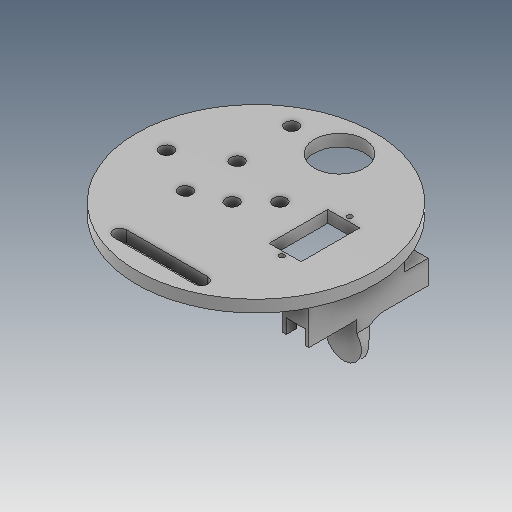
# Autodesk Inventor part: EndEffectorPlate
Saved by Autodesk Inventor 2020.3 (Build 243373000, 373)
## iProperties
Created: 2021-08-11
Part Number: EndEffectorPlate
Material: ABS Plastic
Document SubType Name: Modeling
Designer: justi
Density: 1.06 g/cm^3
Appearance: Smooth - Medium Gray
Mass: 42.5954 g
Surface Area: 204.332 cm^2
Volume: 40.1844 cm^3
Author: justi
Autodesk Inventor part; units mm, degrees
ref_plane "YZ Plane" through (0, 0, 0) normal (1, 0, 0) x (0, 1, 0)
ref_plane "XZ Plane" through (0, 0, 0) normal (0, 1, 0) x (-1, 0, 0)
ref_plane "XY Plane" through (0, 0, 0) normal (0, 0, 1) x (1, 0, 0)
sketch "Sketch1" plane through (0, 0, 0) normal (0, 1, 0) x (-1, 0, 0)
  circle A0 centre (0, 0) radius 50
  dimension "d0" = 100
  constraints: 1 centre point, 1 coincident
  measures "d0" diameter of A0
extrude "Extrusion1" add sketch "Sketch1" along normal mid plane 5
sketch "Sketch2" plane through (0, 2.5, 0) normal (0, 1, 0) x (1, 0, 0)
  line L0 (-5, 5) -> (5, 5) construction
  line L1 (5, 5) -> (5, -5) construction
  line L2 (5, -5) -> (-5, -5) construction
  line L3 (-5, -5) -> (-5, 5) construction
  line L4 (-5, 5) -> (5, -5) construction
  line L5 (5, 5) -> (-5, -5) construction
  circle A0 centre (5, 5) radius 2.75
  circle A1 centre (-5, -5) radius 2.75
  point P0 (0, 0)
  dimension "d77" = 10
  dimension "d78" = 10
  dimension "d80" = 5.5
  dimension "d81" = 5.5
  constraints: 12 end point, 2 centre point, 2 coincident, 2 midpoint, 2 parallel, 1 horizontal, 1 perpendicular
  measures "d77" distance of L1.end L2.end
  measures "d78" distance of L0.end L1.end
  measures "d80" diameter of A0
  measures "d81" diameter of A1
extrude "Extrusion2" cut sketch "Sketch2" against normal blind 10
sketch "Sketch3" plane through (0, 2.5, 0) normal (0, 1, 0) x (1, 0, 0)
  line L0 (0, 0) -> (25, 0) construction
  line L1 (18.8, -11.3) -> (31.2, -11.3)
  line L2 (31.2, -11.3) -> (31.2, 11.3)
  line L3 (31.2, 11.3) -> (18.8, 11.3)
  line L4 (18.8, 11.3) -> (18.8, -11.3)
  line L5 (18.8, -11.3) -> (31.2, 11.3) construction
  line L6 (31.2, -11.3) -> (18.8, 11.3) construction
  line L7 (25, 0) -> (25, 14.25) construction
  line L8 (25, 0) -> (25, -14.25) construction
  circle A0 centre (25, 14.25) radius 1.1
  circle A1 centre (25, -14.25) radius 1.1
  dimension "d9" = 25
  dimension "d10" = 12.4
  dimension "d11" = 22.6
  dimension "d21" = 14.25
  dimension "d22" = 14.25
  dimension "d23" = 2.2
  dimension "d24" = 2.2
  constraints: 18 end point, 2 centre point, 2 coincident, 2 horizontal, 2 midpoint, 2 parallel, 2 vertical, 1 perpendicular
  measures "d9" distance of L0.start L0.end
  measures "d10" distance of L3.end L2.end
  measures "d11" distance of L2.end L1.end
  measures "d21" distance of L0.end L7.end
  measures "d22" distance of L0.end L8.end
  measures "d23" diameter of A0
  measures "d24" diameter of A1
extrude "Extrusion3" cut sketch "Sketch3" against normal blind 10
sketch "Sketch5" plane through (0, -2.5, 0) normal (0, -1, 0) x (1, 0, 0)
  line L0 (31.2, -11.3) -> (33.7, -11.3)
  line L1 (33.7, -11.3) -> (33.7, 11.3)
  line L2 (33.7, 11.3) -> (31.2, 11.3)
  line L3 (31.2, 11.3) -> (31.2, -11.3)
  line L4 (31.2, -11.3) -> (31.2, 11.3) construction
  line L5 (31.2, 0) -> (39.7, 0) construction
  line L6 (39.7, 0) -> (39.7, -20) construction
  line L7 (39.7, -20) -> (31.2, -20)
  line L8 (31.2, -20) -> (31.2, 20)
  line L9 (31.2, 20) -> (39.7, 20)
  line L10 (39.7, 20) -> (39.7, -20)
  line L11 (33.7, -11.3) -> (33.7, -20)
  line L12 (33.7, 11.3) -> (33.7, 20)
  point P0 (0, 0)
  point P1 (31.2, 11.3)
  dimension "d34" = 2.5
  dimension "d35" = 8.5
  dimension "d36" = 20
  dimension "d37" = 40
  constraints: 24 end point, 4 parallel, 4 perpendicular, 3 horizontal, 2 point on line, 1 midpoint, 1 vertical
  measures "d34" distance of L2.end L1.end
  measures "d35" distance of L5.start L5.end
  measures "d36" distance of L5.end L6.end
  measures "d37" distance of L7.end L8.end
extrude "Extrusion5" add sketch "Sketch5" along normal blind 11.8 contours L1 L12 L9 L10 L7 L11
sketch "Sketch6" plane through (0, -2.5, 0) normal (0, -1, 0) x (1, 0, 0)
  line L0 (31.2, -11.3) -> (31.2, 11.3) projected
  line L1 (31.2, 0) -> (33.7, 0)
  line L2 (33.7, 0) -> (33.7, -20)
  line L3 (33.7, -20) -> (31.2, -20)
  line L4 (31.2, -20) -> (31.2, 0)
  line L5 (39.7, 20) -> (33.7, 20) projected
  line L6 (31.2, 0) -> (33.7, 0)
  line L7 (33.7, 0) -> (33.7, 20)
  line L8 (33.7, 20) -> (31.2, 20)
  line L9 (31.2, 20) -> (31.2, 0)
  line L10 (18.8, 11.3) -> (31.2, 11.3) projected
  line L11 (31.2, 11.3) -> (33.7, 11.3)
  line L12 (33.7, -20) -> (33.7, 20) projected
  line L13 (39.7, 20) -> (42.2, 20)
  line L14 (42.2, 20) -> (42.2, -20)
  line L15 (42.2, -20) -> (39.7, -20)
  line L16 (39.7, -20) -> (39.7, 20)
  line L17 (31.2, -15.9678) -> (33.7, -15.9678)
  point P0 (0, 0)
  point P1 (31.2, 11.3)
  dimension "d40" = 2.5
  constraints: 28 end point, 6 parallel, 5 perpendicular, 3 horizontal, 3 point on line, 1 midpoint
  measures "d40" distance of L14.end L15.end
extrude "Extrusion6" add sketch "Sketch6" along normal blind 16.8 contours L13 L14 L15 L16 | L17 L2 L3 L4 | L9 L8 L7 L11
sketch "Sketch7" plane through (0, -19.3, 0) normal (0, -1, 0) x (1, 0, 0)
  line L0 (42.2, -20) -> (31.2, -20) projected
  line L1 (31.2, -20) -> (42.2, -20)
  line L2 (42.2, -20) -> (42.2, 0)
  line L3 (42.2, 0) -> (31.2, 0)
  line L4 (31.2, 0) -> (31.2, -20)
  point P0 (0, 0)
  constraints: 8 end point, 2 parallel, 1 horizontal, 1 perpendicular
extrude "Extrusion7" add sketch "Sketch7" along normal blind 2.5
sketch "Sketch8" plane through (31.2, -19.3, 0) normal (0, 0, 1) x (1, 0, 0)
  line L0 (0, -2.5) -> (11, -2.5) construction
  line L1 (5.5, -2.5) -> (5.5, -10) construction
  circle A0 centre (5.5, -10) radius 7.5
  line L2 (0, 16.8) -> (0, -2.5) construction
  line L3 (11, 16.8) -> (11, -2.5) projected
  line L4 (11, -2.5) -> (11, -4.901)
  line L5 (0, -2.5) -> (0, -4.901)
  line L6 (11, -2.5) -> (0, -2.5)
  point P0 (-31.2, 19.3)
  dimension "d45" = 7.5
  constraints: 8 end point, 3 point on circle, 2 collinear, 1 centre point, 1 coincident, 1 midpoint, 1 parallel, 1 vertical
  measures "d45" distance of L1.start L1.end
extrude "Extrusion8" add sketch "Sketch8" against normal blind 3
fillet "Fillet1" radius 8.25 1 edges at (36.7, -21.8, -3)
sketch "Sketch9" plane through (42.2, -2.5, -20) normal (0, 0, -1) x (-1, 0, 0)
  line L0 (11, -16.8) -> (8.5, -16.8) projected
  line L1 (8.5, -16.8) -> (2.5, -16.8)
  line L2 (2.5, -16.8) -> (2.5, -11.8)
  line L3 (2.5, -11.8) -> (8.5, -11.8)
  line L4 (8.5, -11.8) -> (8.5, -16.8)
  line L5 (11, 0) -> (11, -19.3) projected
  line L6 (0, 0) -> (0, -19.3) projected
  line L7 (11, -19.3) -> (0, -19.3)
  line L8 (0, -19.3) -> (0, -9.35)
  line L9 (0, -9.35) -> (11, -9.35)
  line L10 (11, -9.35) -> (11, -19.3)
  point P0 (42.2, 2.5)
  dimension "d49" = 9.95
  constraints: 16 end point, 4 parallel, 2 horizontal, 2 perpendicular, 1 point on line
  measures "d49" distance of L7.end L8.end
extrude "Extrusion9" add sketch "Sketch9" along normal blind 10
sketch "Sketch12" plane through (0, 2.5, 0) normal (0, 1, 0) x (1, 0, 0)
  circle A0 centre (-25, 0) radius 12.5 construction
  line L0 (-25, 0) -> (-18.75, -10.8253) construction
  line L1 (-25, 0) -> (-37.5, 0) construction
  line L2 (-25, 0) -> (-18.75, 10.8253) construction
  circle A1 centre (-37.5, 0) radius 2.75
  circle A2 centre (-18.75, 10.8253) radius 2.75
  circle A3 centre (-18.75, -10.8253) radius 2.75
  point P0 (0, 0)
  dimension "d64" = 25
  dimension "d65" = 120
  dimension "d67" = 5.5
  dimension "d68" = 5.5
  dimension "d69" = 5.5
  dimension "d70" = 25
  constraints: 6 end point, 4 centre point, 3 coincident, 1 equal length
  measures "d64" diameter of A0
  measures "d65" angle of L1 L0
  measures "d67" diameter of A1
  measures "d68" diameter of A2
  measures "d69" diameter of A3
  measures "d70" distance of point (0, 0) L0.start
extrude "Extrusion12" cut sketch "Sketch12" against normal blind 10
sketch "Sketch13" plane through (0, -2.5, 0) normal (0, -1, 0) x (1, 0, 0)
  line L0 (0, 0) -> (0, -35) construction
  circle A0 centre (0, -35) radius 10.5
  dimension "d73" = 35
  dimension "d74" = 21
  constraints: 2 end point, 1 centre point, 1 coincident, 1 vertical
  measures "d73" distance of L0.start L0.end
  measures "d74" diameter of A0
extrude "Extrusion13" cut sketch "Sketch13" against normal blind 10
sketch "Sketch14" plane through (31.2, -2.5, 20) normal (0, 0, 1) x (1, 0, 0)
  line L0 (8.5, -16.8) -> (2.5, -16.8)
  line L1 (2.5, -16.8) -> (2.5, -11.8)
  line L2 (2.5, -11.8) -> (8.5, -11.8)
  line L3 (8.5, -11.8) -> (8.5, -16.8)
  line L4 (1.5, -17.8) -> (9.5, -17.8)
  line L5 (9.5, -17.8) -> (9.5, -10.8)
  line L6 (9.5, -10.8) -> (1.5, -10.8)
  line L7 (1.5, -10.8) -> (1.5, -17.8)
  point P0 (-31.2, 2.5)
  dimension "d83" = 1
  constraints: 16 end point, 4 parallel, 2 perpendicular, 1 horizontal, 3 other
  measures "d83" distance between parallel lines of L0 L4
extrude "Extrusion14" cut sketch "Sketch14" against normal through all
sketch "Sketch17" plane through (0, -2.5, 0) normal (0, -1, 0) x (1, 0, 0)
  line L0 (0, 0) -> (0, 40) construction
  line L1 (-17, 40) -> (17, 40) construction
  line L2 (-17, 37.25) -> (17, 37.25)
  line L3 (17, 42.75) -> (-17, 42.75)
  arc A0 (-17, 42.75) -> (-17, 37.25) centre (-17, 40) ccw
  arc A1 (17, 37.25) -> (17, 42.75) centre (17, 40) ccw
  dimension "d104" = 17
  dimension "d105" = 5.5
  constraints: 10 end point, 4 point on circle, 4 tangent, 2 centre point, 1 midpoint, 1 parallel, 1 perpendicular, 1 vertical
  measures "d104" distance of L0.end L1.end
  measures "d105" diameter of A1
extrude "Extrusion15" cut sketch "Sketch17" against normal through all
sketch "Sketch18" plane through (0, -2.5, 0) normal (0, -1, 0) x (1, 0, 0)
  line L0 (31.2, 20) -> (31.2, 11.3) projected
  line L1 (31.2, 11.3) -> (31.2, 12.3)
  line L2 (31.2, 12.3) -> (17.8, 12.3)
  line L3 (17.8, 12.3) -> (31.2, 12.3)
  line L4 (31.2, 12.3) -> (31.2, -12.3)
  line L5 (31.2, -12.3) -> (17.8, -12.3)
  line L6 (17.8, -12.3) -> (17.8, 12.3)
  point P0 (0, 0)
  dimension "d93" = 1
  dimension "d94" = 13.4
  dimension "d95" = 24.6
  constraints: 12 end point, 2 parallel, 2 perpendicular, 1 horizontal, 1 point on line
  measures "d93" distance of L0.end L1.end
  measures "d94" distance of L1.end L2.end
  measures "d95" distance of L3.end L4.end
extrude "Extrusion16" cut sketch "Sketch18" against normal blind 10
sketch "Sketch19" plane through (31.2, -19.3, 11.3) normal (-1, 0, 0) x (0, 0, 1)
  line L0 (-27.2678, 6) -> (0, 6) projected
  line L1 (8.7, 0) -> (0, 0) projected
  line L2 (0, 6) -> (4.35, 6)
  line L3 (4.35, 6) -> (4.35, 0)
  line L4 (4.35, 0) -> (0, 0)
  line L5 (0, 0) -> (0, 6)
  point P0 (-11.3, 19.3)
  constraints: 8 end point, 2 parallel, 1 horizontal, 1 midpoint, 1 perpendicular
extrude "Extrusion17" cut sketch "Sketch19" against normal up to surface (1.5 mm away)
sketch "Sketch22" plane through (0, 2.5, 0) normal (0, 1, 0) x (1, 0, 0)
  circle A0 centre (0, 35) radius 10.5 projected
  line L0 (0, 35) -> (-20, 35) construction
  circle A1 centre (-20, 35) radius 2.75
  point P0 (0, 0)
  dimension "d100" = 20
  dimension "d101" = 5.5
  constraints: 2 coincident, 2 end point, 1 centre point, 1 horizontal
  measures "d100" distance of L0.start L0.end
  measures "d101" diameter of A1
extrude "Extrusion18" cut sketch "Sketch22" against normal blind 10 contours A1
equation "\"d80\" = d82"
equation "\"d81\" = d82"
equation "\"d82\" = 5.5"
body "Solid1"
